Autodesk Fusion 360 part; units mm, degrees
(part 2 of 4)
  line L902 (-16.4615, 144.9808) -> (-16.4615, 149.9808)
  line L903 (-16.4615, 149.9808) -> (-20.7917, 152.4808)
  line L904 (-31.4519, 152.4808) -> (-35.782, 149.9808)
  line L905 (-35.782, 149.9808) -> (-35.782, 144.9808)
  line L906 (-35.782, 144.9808) -> (-31.4519, 142.4808)
  line L907 (-31.4519, 142.4808) -> (-27.1218, 144.9808)
  line L908 (-27.1218, 144.9808) -> (-27.1218, 149.9808)
  line L909 (-27.1218, 149.9808) -> (-31.4519, 152.4808)
  line L910 (-42.1122, 152.4808) -> (-46.4423, 149.9808)
  line L911 (-46.4423, 149.9808) -> (-46.4423, 144.9808)
  line L912 (-46.4423, 144.9808) -> (-42.1122, 142.4808)
  line L913 (-42.1122, 142.4808) -> (-37.782, 144.9808)
  line L914 (-37.782, 144.9808) -> (-37.782, 149.9808)
  line L915 (-37.782, 149.9808) -> (-42.1122, 152.4808)
  line L916 (48.5, 161.7128) -> (44.1699, 159.2128)
  line L917 (44.1699, 159.2128) -> (44.1699, 154.2128)
  line L918 (44.1699, 154.2128) -> (48.5, 151.7128)
  line L919 (48.5, 151.7128) -> (52.8301, 154.2128)
  line L920 (52.8301, 154.2128) -> (52.8301, 159.2128)
  line L921 (52.8301, 159.2128) -> (48.5, 161.7128)
  line L922 (37.8397, 161.7128) -> (33.5096, 159.2128)
  line L923 (33.5096, 159.2128) -> (33.5096, 154.2128)
  line L924 (33.5096, 154.2128) -> (37.8397, 151.7128)
  line L925 (37.8397, 151.7128) -> (42.1699, 154.2128)
  line L926 (42.1699, 154.2128) -> (42.1699, 159.2128)
  line L927 (42.1699, 159.2128) -> (37.8397, 161.7128)
  line L928 (27.1795, 161.7128) -> (22.8494, 159.2128)
  line L929 (22.8494, 159.2128) -> (22.8494, 154.2128)
  line L930 (22.8494, 154.2128) -> (27.1795, 151.7128)
  line L931 (27.1795, 151.7128) -> (31.5096, 154.2128)
  line L932 (31.5096, 154.2128) -> (31.5096, 159.2128)
  line L933 (31.5096, 159.2128) -> (27.1795, 161.7128)
  line L934 (16.5192, 161.7128) -> (12.1891, 159.2128)
  line L935 (12.1891, 159.2128) -> (12.1891, 154.2128)
  line L936 (12.1891, 154.2128) -> (16.5192, 151.7128)
  line L937 (16.5192, 151.7128) -> (20.8494, 154.2128)
  line L938 (20.8494, 154.2128) -> (20.8494, 159.2128)
  line L939 (20.8494, 159.2128) -> (16.5192, 161.7128)
  line L940 (5.859, 161.7128) -> (1.5289, 159.2128)
  line L941 (1.5289, 159.2128) -> (1.5289, 154.2128)
  line L942 (1.5289, 154.2128) -> (5.859, 151.7128)
  line L943 (5.859, 151.7128) -> (10.1891, 154.2128)
  line L944 (10.1891, 154.2128) -> (10.1891, 159.2128)
  line L945 (10.1891, 159.2128) -> (5.859, 161.7128)
  line L946 (-4.8013, 161.7128) -> (-9.1314, 159.2128)
  line L947 (-9.1314, 159.2128) -> (-9.1314, 154.2128)
  line L948 (-9.1314, 154.2128) -> (-4.8013, 151.7128)
  line L949 (-4.8013, 151.7128) -> (-0.4711, 154.2128)
  line L950 (-0.4711, 154.2128) -> (-0.4711, 159.2128)
  line L951 (-0.4711, 159.2128) -> (-4.8013, 161.7128)
  line L952 (-15.4615, 161.7128) -> (-19.7917, 159.2128)
  line L953 (-19.7917, 159.2128) -> (-19.7917, 154.2128)
  line L954 (-19.7917, 154.2128) -> (-15.4615, 151.7128)
  line L955 (-15.4615, 151.7128) -> (-11.1314, 154.2128)
  line L956 (-11.1314, 154.2128) -> (-11.1314, 159.2128)
  line L957 (-11.1314, 159.2128) -> (-15.4615, 161.7128)
  line L958 (-26.1218, 161.7128) -> (-30.4519, 159.2128)
  line L959 (-30.4519, 159.2128) -> (-30.4519, 154.2128)
  line L960 (-30.4519, 154.2128) -> (-26.1218, 151.7128)
  line L961 (-26.1218, 151.7128) -> (-21.7917, 154.2128)
  line L962 (-21.7917, 154.2128) -> (-21.7917, 159.2128)
  line L963 (-21.7917, 159.2128) -> (-26.1218, 161.7128)
  line L964 (-36.782, 161.7128) -> (-41.1122, 159.2128)
  line L965 (-41.1122, 159.2128) -> (-41.1122, 154.2128)
  line L966 (-41.1122, 154.2128) -> (-36.782, 151.7128)
  line L967 (-36.782, 151.7128) -> (-32.4519, 154.2128)
  line L968 (-32.4519, 154.2128) -> (-32.4519, 159.2128)
  line L969 (-32.4519, 159.2128) -> (-36.782, 161.7128)
  line L970 (-47.4423, 161.7128) -> (-51.7724, 159.2128)
  line L971 (-51.7724, 159.2128) -> (-51.7724, 154.2128)
  line L972 (-51.7724, 154.2128) -> (-47.4423, 151.7128)
  line L973 (-47.4423, 151.7128) -> (-43.1122, 154.2128)
  line L974 (-43.1122, 154.2128) -> (-43.1122, 159.2128)
  line L975 (-43.1122, 159.2128) -> (-47.4423, 161.7128)
  line L976 (43.1699, 170.9449) -> (38.8397, 168.4449)
  line L977 (38.8397, 168.4449) -> (38.8397, 163.4449)
  line L978 (38.8397, 163.4449) -> (43.1699, 160.9449)
  line L979 (43.1699, 160.9449) -> (47.5, 163.4449)
  line L980 (47.5, 163.4449) -> (47.5, 168.4449)
  line L981 (47.5, 168.4449) -> (43.1699, 170.9449)
  line L982 (32.5096, 170.9449) -> (28.1795, 168.4449)
  line L983 (28.1795, 168.4449) -> (28.1795, 163.4449)
  line L984 (28.1795, 163.4449) -> (32.5096, 160.9449)
  line L985 (32.5096, 160.9449) -> (36.8397, 163.4449)
  line L986 (36.8397, 163.4449) -> (36.8397, 168.4449)
  line L987 (36.8397, 168.4449) -> (32.5096, 170.9449)
  line L988 (21.8494, 170.9449) -> (17.5192, 168.4449)
  line L989 (17.5192, 168.4449) -> (17.5192, 163.4449)
  line L990 (17.5192, 163.4449) -> (21.8494, 160.9449)
  line L991 (21.8494, 160.9449) -> (26.1795, 163.4449)
  line L992 (26.1795, 163.4449) -> (26.1795, 168.4449)
  line L993 (26.1795, 168.4449) -> (21.8494, 170.9449)
  line L994 (11.1891, 170.9449) -> (6.859, 168.4449)
  line L995 (6.859, 168.4449) -> (6.859, 163.4449)
  line L996 (6.859, 163.4449) -> (11.1891, 160.9449)
  line L997 (11.1891, 160.9449) -> (15.5192, 163.4449)
  line L998 (15.5192, 163.4449) -> (15.5192, 168.4449)
  line L999 (15.5192, 168.4449) -> (11.1891, 170.9449)
  line L1000 (0.5289, 170.9449) -> (-3.8013, 168.4449)
  line L1001 (-3.8013, 168.4449) -> (-3.8013, 163.4449)
  line L1002 (-3.8013, 163.4449) -> (0.5289, 160.9449)
  line L1003 (0.5289, 160.9449) -> (4.859, 163.4449)
  line L1004 (4.859, 163.4449) -> (4.859, 168.4449)
  line L1005 (4.859, 168.4449) -> (0.5289, 170.9449)
  line L1006 (-10.1314, 170.9449) -> (-14.4615, 168.4449)
  line L1007 (-14.4615, 168.4449) -> (-14.4615, 163.4449)
  line L1008 (-14.4615, 163.4449) -> (-10.1314, 160.9449)
  line L1009 (-10.1314, 160.9449) -> (-5.8013, 163.4449)
  line L1010 (-5.8013, 163.4449) -> (-5.8013, 168.4449)
  line L1011 (-5.8013, 168.4449) -> (-10.1314, 170.9449)
  line L1012 (-20.7917, 170.9449) -> (-25.1218, 168.4449)
  line L1013 (-25.1218, 168.4449) -> (-25.1218, 163.4449)
  line L1014 (-25.1218, 163.4449) -> (-20.7917, 160.9449)
  line L1015 (-20.7917, 160.9449) -> (-16.4615, 163.4449)
  line L1016 (-16.4615, 163.4449) -> (-16.4615, 168.4449)
  line L1017 (-16.4615, 168.4449) -> (-20.7917, 170.9449)
  line L1018 (-31.4519, 170.9449) -> (-35.782, 168.4449)
  line L1019 (-35.782, 168.4449) -> (-35.782, 163.4449)
  line L1020 (-35.782, 163.4449) -> (-31.4519, 160.9449)
  line L1021 (-31.4519, 160.9449) -> (-27.1218, 163.4449)
  line L1022 (-27.1218, 163.4449) -> (-27.1218, 168.4449)
  line L1023 (-27.1218, 168.4449) -> (-31.4519, 170.9449)
  line L1024 (-42.1122, 170.9449) -> (-46.4423, 168.4449)
  line L1025 (-46.4423, 168.4449) -> (-46.4423, 163.4449)
  line L1026 (-46.4423, 163.4449) -> (-42.1122, 160.9449)
  line L1027 (-42.1122, 160.9449) -> (-37.782, 163.4449)
  line L1028 (-37.782, 163.4449) -> (-37.782, 168.4449)
  line L1029 (-37.782, 168.4449) -> (-42.1122, 170.9449)
  line L1030 (48.5, 180.1769) -> (44.1699, 177.6769)
  line L1031 (44.1699, 177.6769) -> (44.1699, 172.6769)
  line L1032 (44.1699, 172.6769) -> (48.5, 170.1769)
  line L1033 (48.5, 170.1769) -> (52.8301, 172.6769)
  line L1034 (52.8301, 172.6769) -> (52.8301, 177.6769)
  line L1035 (52.8301, 177.6769) -> (48.5, 180.1769)
  line L1036 (37.8397, 180.1769) -> (33.5096, 177.6769)
  line L1037 (33.5096, 177.6769) -> (33.5096, 172.6769)
  line L1038 (33.5096, 172.6769) -> (37.8397, 170.1769)
  line L1039 (37.8397, 170.1769) -> (42.1699, 172.6769)
  line L1040 (42.1699, 172.6769) -> (42.1699, 177.6769)
  line L1041 (42.1699, 177.6769) -> (37.8397, 180.1769)
  line L1042 (27.1795, 180.1769) -> (22.8494, 177.6769)
  line L1043 (22.8494, 177.6769) -> (22.8494, 172.6769)
  line L1044 (22.8494, 172.6769) -> (27.1795, 170.1769)
  line L1045 (27.1795, 170.1769) -> (31.5096, 172.6769)
  line L1046 (31.5096, 172.6769) -> (31.5096, 177.6769)
  line L1047 (31.5096, 177.6769) -> (27.1795, 180.1769)
  line L1048 (16.5192, 180.1769) -> (12.1891, 177.6769)
  line L1049 (12.1891, 177.6769) -> (12.1891, 172.6769)
  line L1050 (12.1891, 172.6769) -> (16.5192, 170.1769)
  line L1051 (16.5192, 170.1769) -> (20.8494, 172.6769)
  line L1052 (20.8494, 172.6769) -> (20.8494, 177.6769)
  line L1053 (20.8494, 177.6769) -> (16.5192, 180.1769)
  line L1054 (5.859, 180.1769) -> (1.5289, 177.6769)
  line L1055 (1.5289, 177.6769) -> (1.5289, 172.6769)
  line L1056 (1.5289, 172.6769) -> (5.859, 170.1769)
  line L1057 (5.859, 170.1769) -> (10.1891, 172.6769)
  line L1058 (10.1891, 172.6769) -> (10.1891, 177.6769)
  line L1059 (10.1891, 177.6769) -> (5.859, 180.1769)
  line L1060 (-4.8013, 180.1769) -> (-9.1314, 177.6769)
  line L1061 (-9.1314, 177.6769) -> (-9.1314, 172.6769)
  line L1062 (-9.1314, 172.6769) -> (-4.8013, 170.1769)
  line L1063 (-4.8013, 170.1769) -> (-0.4711, 172.6769)
  line L1064 (-0.4711, 172.6769) -> (-0.4711, 177.6769)
  line L1065 (-0.4711, 177.6769) -> (-4.8013, 180.1769)
  line L1066 (-15.4615, 180.1769) -> (-19.7917, 177.6769)
  line L1067 (-19.7917, 177.6769) -> (-19.7917, 172.6769)
  line L1068 (-19.7917, 172.6769) -> (-15.4615, 170.1769)
  line L1069 (-15.4615, 170.1769) -> (-11.1314, 172.6769)
  line L1070 (-11.1314, 172.6769) -> (-11.1314, 177.6769)
  line L1071 (-11.1314, 177.6769) -> (-15.4615, 180.1769)
  line L1072 (-26.1218, 180.1769) -> (-30.4519, 177.6769)
  line L1073 (-30.4519, 177.6769) -> (-30.4519, 172.6769)
  line L1074 (-30.4519, 172.6769) -> (-26.1218, 170.1769)
  line L1075 (-26.1218, 170.1769) -> (-21.7917, 172.6769)
  line L1076 (-21.7917, 172.6769) -> (-21.7917, 177.6769)
  line L1077 (-21.7917, 177.6769) -> (-26.1218, 180.1769)
  line L1078 (-36.782, 180.1769) -> (-41.1122, 177.6769)
  line L1079 (-41.1122, 177.6769) -> (-41.1122, 172.6769)
  line L1080 (-41.1122, 172.6769) -> (-36.782, 170.1769)
  line L1081 (-36.782, 170.1769) -> (-32.4519, 172.6769)
  line L1082 (-32.4519, 172.6769) -> (-32.4519, 177.6769)
  line L1083 (-32.4519, 177.6769) -> (-36.782, 180.1769)
  line L1084 (-47.4423, 180.1769) -> (-51.7724, 177.6769)
  line L1085 (-51.7724, 177.6769) -> (-51.7724, 172.6769)
  line L1086 (-51.7724, 172.6769) -> (-47.4423, 170.1769)
  line L1087 (-47.4423, 170.1769) -> (-43.1122, 172.6769)
  line L1088 (-43.1122, 172.6769) -> (-43.1122, 177.6769)
  line L1089 (-43.1122, 177.6769) -> (-47.4423, 180.1769)
  line L1090 (43.1699, 189.409) -> (38.8397, 186.909)
  line L1091 (38.8397, 186.909) -> (38.8397, 181.909)
  line L1092 (38.8397, 181.909) -> (43.1699, 179.409)
  line L1093 (43.1699, 179.409) -> (47.5, 181.909)
  line L1094 (47.5, 181.909) -> (47.5, 186.909)
  line L1095 (47.5, 186.909) -> (43.1699, 189.409)
  line L1096 (32.5096, 189.409) -> (28.1795, 186.909)
  line L1097 (28.1795, 186.909) -> (28.1795, 181.909)
  line L1098 (28.1795, 181.909) -> (32.5096, 179.409)
  line L1099 (32.5096, 179.409) -> (36.8397, 181.909)
  line L1100 (36.8397, 181.909) -> (36.8397, 186.909)
  line L1101 (36.8397, 186.909) -> (32.5096, 189.409)
  line L1102 (21.8494, 189.409) -> (17.5192, 186.909)
  line L1103 (17.5192, 186.909) -> (17.5192, 181.909)
  line L1104 (17.5192, 181.909) -> (21.8494, 179.409)
  line L1105 (21.8494, 179.409) -> (26.1795, 181.909)
  line L1106 (26.1795, 181.909) -> (26.1795, 186.909)
  line L1107 (26.1795, 186.909) -> (21.8494, 189.409)
  line L1108 (11.1891, 189.409) -> (6.859, 186.909)
  line L1109 (6.859, 186.909) -> (6.859, 181.909)
  line L1110 (6.859, 181.909) -> (11.1891, 179.409)
  line L1111 (11.1891, 179.409) -> (15.5192, 181.909)
  line L1112 (15.5192, 181.909) -> (15.5192, 186.909)
  line L1113 (15.5192, 186.909) -> (11.1891, 189.409)
  line L1114 (0.5289, 189.409) -> (-3.8013, 186.909)
  line L1115 (-3.8013, 186.909) -> (-3.8013, 181.909)
  line L1116 (-3.8013, 181.909) -> (0.5289, 179.409)
  line L1117 (0.5289, 179.409) -> (4.859, 181.909)
  line L1118 (4.859, 181.909) -> (4.859, 186.909)
  line L1119 (4.859, 186.909) -> (0.5289, 189.409)
  line L1120 (-10.1314, 189.409) -> (-14.4615, 186.909)
  line L1121 (-14.4615, 186.909) -> (-14.4615, 181.909)
  line L1122 (-14.4615, 181.909) -> (-10.1314, 179.409)
  line L1123 (-10.1314, 179.409) -> (-5.8013, 181.909)
  line L1124 (-5.8013, 181.909) -> (-5.8013, 186.909)
  line L1125 (-5.8013, 186.909) -> (-10.1314, 189.409)
  line L1126 (-20.7917, 189.409) -> (-25.1218, 186.909)
  line L1127 (-25.1218, 186.909) -> (-25.1218, 181.909)
  line L1128 (-25.1218, 181.909) -> (-20.7917, 179.409)
  line L1129 (-20.7917, 179.409) -> (-16.4615, 181.909)
  line L1130 (-16.4615, 181.909) -> (-16.4615, 186.909)
  line L1131 (-16.4615, 186.909) -> (-20.7917, 189.409)
  line L1132 (-31.4519, 189.409) -> (-35.782, 186.909)
  line L1133 (-35.782, 186.909) -> (-35.782, 181.909)
  line L1134 (-35.782, 181.909) -> (-31.4519, 179.409)
  line L1135 (-31.4519, 179.409) -> (-27.1218, 181.909)
  line L1136 (-27.1218, 181.909) -> (-27.1218, 186.909)
  line L1137 (-27.1218, 186.909) -> (-31.4519, 189.409)
  line L1138 (-42.1122, 189.409) -> (-46.4423, 186.909)
  line L1139 (-46.4423, 186.909) -> (-46.4423, 181.909)
  line L1140 (-46.4423, 181.909) -> (-42.1122, 179.409)
  line L1141 (-42.1122, 179.409) -> (-37.782, 181.909)
  line L1142 (-37.782, 181.909) -> (-37.782, 186.909)
  line L1143 (-37.782, 186.909) -> (-42.1122, 189.409)
  line L1144 (48.5, 198.641) -> (44.1699, 196.141)
  line L1145 (44.1699, 196.141) -> (44.1699, 191.141)
  line L1146 (44.1699, 191.141) -> (48.5, 188.641)
  line L1147 (48.5, 188.641) -> (52.8301, 191.141)
  line L1148 (52.8301, 191.141) -> (52.8301, 196.141)
  line L1149 (52.8301, 196.141) -> (48.5, 198.641)
  line L1150 (37.8397, 198.641) -> (33.5096, 196.141)
  line L1151 (33.5096, 196.141) -> (33.5096, 191.141)
  line L1152 (33.5096, 191.141) -> (37.8397, 188.641)
  line L1153 (37.8397, 188.641) -> (42.1699, 191.141)
  line L1154 (42.1699, 191.141) -> (42.1699, 196.141)
  line L1155 (42.1699, 196.141) -> (37.8397, 198.641)
  line L1156 (27.1795, 198.641) -> (22.8494, 196.141)
  line L1157 (22.8494, 196.141) -> (22.8494, 191.141)
  line L1158 (22.8494, 191.141) -> (27.1795, 188.641)
  line L1159 (27.1795, 188.641) -> (31.5096, 191.141)
  line L1160 (31.5096, 191.141) -> (31.5096, 196.141)
  line L1161 (31.5096, 196.141) -> (27.1795, 198.641)
  line L1162 (16.5192, 198.641) -> (12.1891, 196.141)
  line L1163 (12.1891, 196.141) -> (12.1891, 191.141)
  line L1164 (12.1891, 191.141) -> (16.5192, 188.641)
  line L1165 (16.5192, 188.641) -> (20.8494, 191.141)
  line L1166 (20.8494, 191.141) -> (20.8494, 196.141)
  line L1167 (20.8494, 196.141) -> (16.5192, 198.641)
  line L1168 (5.859, 198.641) -> (1.5289, 196.141)
  line L1169 (1.5289, 196.141) -> (1.5289, 191.141)
  line L1170 (1.5289, 191.141) -> (5.859, 188.641)
  line L1171 (5.859, 188.641) -> (10.1891, 191.141)
  line L1172 (10.1891, 191.141) -> (10.1891, 196.141)
  line L1173 (10.1891, 196.141) -> (5.859, 198.641)
  line L1174 (-4.8013, 198.641) -> (-9.1314, 196.141)
  line L1175 (-9.1314, 196.141) -> (-9.1314, 191.141)
  line L1176 (-9.1314, 191.141) -> (-4.8013, 188.641)
  line L1177 (-4.8013, 188.641) -> (-0.4711, 191.141)
  line L1178 (-0.4711, 191.141) -> (-0.4711, 196.141)
  line L1179 (-0.4711, 196.141) -> (-4.8013, 198.641)
  line L1180 (-15.4615, 198.641) -> (-19.7917, 196.141)
  line L1181 (-19.7917, 196.141) -> (-19.7917, 191.141)
  line L1182 (-19.7917, 191.141) -> (-15.4615, 188.641)
  line L1183 (-15.4615, 188.641) -> (-11.1314, 191.141)
  line L1184 (-11.1314, 191.141) -> (-11.1314, 196.141)
  line L1185 (-11.1314, 196.141) -> (-15.4615, 198.641)
  line L1186 (-26.1218, 198.641) -> (-30.4519, 196.141)
  line L1187 (-30.4519, 196.141) -> (-30.4519, 191.141)
  line L1188 (-30.4519, 191.141) -> (-26.1218, 188.641)
  line L1189 (-26.1218, 188.641) -> (-21.7917, 191.141)
  line L1190 (-21.7917, 191.141) -> (-21.7917, 196.141)
  line L1191 (-21.7917, 196.141) -> (-26.1218, 198.641)
  line L1192 (-36.782, 198.641) -> (-41.1122, 196.141)
  line L1193 (-41.1122, 196.141) -> (-41.1122, 191.141)
  line L1194 (-41.1122, 191.141) -> (-36.782, 188.641)
  line L1195 (-36.782, 188.641) -> (-32.4519, 191.141)
  line L1196 (-32.4519, 191.141) -> (-32.4519, 196.141)
  line L1197 (-32.4519, 196.141) -> (-36.782, 198.641)
  line L1198 (-47.4423, 198.641) -> (-51.7724, 196.141)
  line L1199 (-51.7724, 196.141) -> (-51.7724, 191.141)
  line L1200 (-51.7724, 191.141) -> (-47.4423, 188.641)
  line L1201 (-47.4423, 188.641) -> (-43.1122, 191.141)
  line L1202 (-43.1122, 191.141) -> (-43.1122, 196.141)
  line L1203 (-43.1122, 196.141) -> (-47.4423, 198.641)
  line L1204 (43.1699, 207.8731) -> (38.8397, 205.3731)
  line L1205 (38.8397, 205.3731) -> (38.8397, 200.3731)
  line L1206 (38.8397, 200.3731) -> (43.1699, 197.8731)
  line L1207 (43.1699, 197.8731) -> (47.5, 200.3731)
  line L1208 (47.5, 200.3731) -> (47.5, 205.3731)
  line L1209 (47.5, 205.3731) -> (43.1699, 207.8731)
  line L1210 (32.5096, 207.8731) -> (28.1795, 205.3731)
  line L1211 (28.1795, 205.3731) -> (28.1795, 200.3731)
  line L1212 (28.1795, 200.3731) -> (32.5096, 197.8731)
  line L1213 (32.5096, 197.8731) -> (36.8397, 200.3731)
  line L1214 (36.8397, 200.3731) -> (36.8397, 205.3731)
  line L1215 (36.8397, 205.3731) -> (32.5096, 207.8731)
  line L1216 (21.8494, 207.8731) -> (17.5192, 205.3731)
  line L1217 (17.5192, 205.3731) -> (17.5192, 200.3731)
  line L1218 (17.5192, 200.3731) -> (21.8494, 197.8731)
  line L1219 (21.8494, 197.8731) -> (26.1795, 200.3731)
  line L1220 (26.1795, 200.3731) -> (26.1795, 205.3731)
  line L1221 (26.1795, 205.3731) -> (21.8494, 207.8731)
  line L1222 (11.1891, 207.8731) -> (6.859, 205.3731)
  line L1223 (6.859, 205.3731) -> (6.859, 200.3731)
  line L1224 (6.859, 200.3731) -> (11.1891, 197.8731)
  line L1225 (11.1891, 197.8731) -> (15.5192, 200.3731)
  line L1226 (15.5192, 200.3731) -> (15.5192, 205.3731)
  line L1227 (15.5192, 205.3731) -> (11.1891, 207.8731)
  line L1228 (0.5289, 207.8731) -> (-3.8013, 205.3731)
  line L1229 (-3.8013, 205.3731) -> (-3.8013, 200.3731)
  line L1230 (-3.8013, 200.3731) -> (0.5289, 197.8731)
  line L1231 (0.5289, 197.8731) -> (4.859, 200.3731)
  line L1232 (4.859, 200.3731) -> (4.859, 205.3731)
  line L1233 (4.859, 205.3731) -> (0.5289, 207.8731)
  line L1234 (-10.1314, 207.8731) -> (-14.4615, 205.3731)
  line L1235 (-14.4615, 205.3731) -> (-14.4615, 200.3731)
  line L1236 (-14.4615, 200.3731) -> (-10.1314, 197.8731)
  line L1237 (-10.1314, 197.8731) -> (-5.8013, 200.3731)
  line L1238 (-5.8013, 200.3731) -> (-5.8013, 205.3731)
  line L1239 (-5.8013, 205.3731) -> (-10.1314, 207.8731)
  line L1240 (-20.7917, 207.8731) -> (-25.1218, 205.3731)
  line L1241 (-25.1218, 205.3731) -> (-25.1218, 200.3731)
  line L1242 (-25.1218, 200.3731) -> (-20.7917, 197.8731)
  line L1243 (-20.7917, 197.8731) -> (-16.4615, 200.3731)
  line L1244 (-16.4615, 200.3731) -> (-16.4615, 205.3731)
  line L1245 (-16.4615, 205.3731) -> (-20.7917, 207.8731)
  line L1246 (-31.4519, 207.8731) -> (-35.782, 205.3731)
  line L1247 (-35.782, 205.3731) -> (-35.782, 200.3731)
  line L1248 (-35.782, 200.3731) -> (-31.4519, 197.8731)
  line L1249 (-31.4519, 197.8731) -> (-27.1218, 200.3731)
  line L1250 (-27.1218, 200.3731) -> (-27.1218, 205.3731)
  line L1251 (-27.1218, 205.3731) -> (-31.4519, 207.8731)
  line L1252 (-42.1122, 207.8731) -> (-46.4423, 205.3731)
  line L1253 (-46.4423, 205.3731) -> (-46.4423, 200.3731)
  line L1254 (-46.4423, 200.3731) -> (-42.1122, 197.8731)
  line L1255 (-42.1122, 197.8731) -> (-37.782, 200.3731)
  line L1256 (-37.782, 200.3731) -> (-37.782, 205.3731)
  line L1257 (-37.782, 205.3731) -> (-42.1122, 207.8731)
  line L1258 (48.5, 217.1051) -> (44.1699, 214.6051)
  line L1259 (44.1699, 214.6051) -> (44.1699, 209.6051)
  line L1260 (44.1699, 209.6051) -> (48.5, 207.1051)
  line L1261 (48.5, 207.1051) -> (52.8301, 209.6051)
  line L1262 (52.8301, 209.6051) -> (52.8301, 214.6051)
  line L1263 (52.8301, 214.6051) -> (48.5, 217.1051)
  line L1264 (37.8397, 217.1051) -> (33.5096, 214.6051)
  line L1265 (33.5096, 214.6051) -> (33.5096, 209.6051)
  line L1266 (33.5096, 209.6051) -> (37.8397, 207.1051)
  line L1267 (37.8397, 207.1051) -> (42.1699, 209.6051)
  line L1268 (42.1699, 209.6051) -> (42.1699, 214.6051)
  line L1269 (42.1699, 214.6051) -> (37.8397, 217.1051)
  line L1270 (27.1795, 217.1051) -> (22.8494, 214.6051)
  line L1271 (22.8494, 214.6051) -> (22.8494, 209.6051)
  line L1272 (22.8494, 209.6051) -> (27.1795, 207.1051)
  line L1273 (27.1795, 207.1051) -> (31.5096, 209.6051)
  line L1274 (31.5096, 209.6051) -> (31.5096, 214.6051)
  line L1275 (31.5096, 214.6051) -> (27.1795, 217.1051)
  line L1276 (16.5192, 217.1051) -> (12.1891, 214.6051)
  line L1277 (12.1891, 214.6051) -> (12.1891, 209.6051)
  line L1278 (12.1891, 209.6051) -> (16.5192, 207.1051)
  line L1279 (16.5192, 207.1051) -> (20.8494, 209.6051)
  line L1280 (20.8494, 209.6051) -> (20.8494, 214.6051)
  line L1281 (20.8494, 214.6051) -> (16.5192, 217.1051)
  line L1282 (5.859, 217.1051) -> (1.5289, 214.6051)
  line L1283 (1.5289, 214.6051) -> (1.5289, 209.6051)
  line L1284 (1.5289, 209.6051) -> (5.859, 207.1051)
  line L1285 (5.859, 207.1051) -> (10.1891, 209.6051)
  line L1286 (10.1891, 209.6051) -> (10.1891, 214.6051)
  line L1287 (10.1891, 214.6051) -> (5.859, 217.1051)
  line L1288 (-4.8013, 217.1051) -> (-9.1314, 214.6051)
  line L1289 (-9.1314, 214.6051) -> (-9.1314, 209.6051)
  line L1290 (-9.1314, 209.6051) -> (-4.8013, 207.1051)
  line L1291 (-4.8013, 207.1051) -> (-0.4711, 209.6051)
  line L1292 (-0.4711, 209.6051) -> (-0.4711, 214.6051)
  line L1293 (-0.4711, 214.6051) -> (-4.8013, 217.1051)
  line L1294 (-15.4615, 217.1051) -> (-19.7917, 214.6051)
  line L1295 (-19.7917, 214.6051) -> (-19.7917, 209.6051)
  line L1296 (-19.7917, 209.6051) -> (-15.4615, 207.1051)
  line L1297 (-15.4615, 207.1051) -> (-11.1314, 209.6051)
  line L1298 (-11.1314, 209.6051) -> (-11.1314, 214.6051)
  line L1299 (-11.1314, 214.6051) -> (-15.4615, 217.1051)
  line L1300 (-26.1218, 217.1051) -> (-30.4519, 214.6051)
  line L1301 (-30.4519, 214.6051) -> (-30.4519, 209.6051)
  line L1302 (-30.4519, 209.6051) -> (-26.1218, 207.1051)
  line L1303 (-26.1218, 207.1051) -> (-21.7917, 209.6051)
  line L1304 (-21.7917, 209.6051) -> (-21.7917, 214.6051)
  line L1305 (-21.7917, 214.6051) -> (-26.1218, 217.1051)
  line L1306 (-36.782, 217.1051) -> (-41.1122, 214.6051)
  line L1307 (-41.1122, 214.6051) -> (-41.1122, 209.6051)
  line L1308 (-41.1122, 209.6051) -> (-36.782, 207.1051)
  line L1309 (-36.782, 207.1051) -> (-32.4519, 209.6051)
  line L1310 (-32.4519, 209.6051) -> (-32.4519, 214.6051)
  line L1311 (-32.4519, 214.6051) -> (-36.782, 217.1051)
  line L1312 (-47.4423, 217.1051) -> (-51.7724, 214.6051)
  line L1313 (-51.7724, 214.6051) -> (-51.7724, 209.6051)
  line L1314 (-51.7724, 209.6051) -> (-47.4423, 207.1051)
  line L1315 (-47.4423, 207.1051) -> (-43.1122, 209.6051)
  line L1316 (-43.1122, 209.6051) -> (-43.1122, 214.6051)
  line L1317 (-43.1122, 214.6051) -> (-47.4423, 217.1051)
  line L1318 (43.1699, 226.3372) -> (38.8397, 223.8372)
  line L1319 (38.8397, 223.8372) -> (38.8397, 218.8372)
  line L1320 (38.8397, 218.8372) -> (43.1699, 216.3372)
  line L1321 (43.1699, 216.3372) -> (47.5, 218.8372)
  line L1322 (47.5, 218.8372) -> (47.5, 223.8372)
  line L1323 (47.5, 223.8372) -> (43.1699, 226.3372)
  line L1324 (32.5096, 226.3372) -> (28.1795, 223.8372)
  line L1325 (28.1795, 223.8372) -> (28.1795, 218.8372)
  line L1326 (28.1795, 218.8372) -> (32.5096, 216.3372)
  line L1327 (32.5096, 216.3372) -> (36.8397, 218.8372)
  line L1328 (36.8397, 218.8372) -> (36.8397, 223.8372)
  line L1329 (36.8397, 223.8372) -> (32.5096, 226.3372)
  line L1330 (21.8494, 226.3372) -> (17.5192, 223.8372)
  line L1331 (17.5192, 223.8372) -> (17.5192, 218.8372)
  line L1332 (17.5192, 218.8372) -> (21.8494, 216.3372)
  line L1333 (21.8494, 216.3372) -> (26.1795, 218.8372)
  line L1334 (26.1795, 218.8372) -> (26.1795, 223.8372)
  line L1335 (26.1795, 223.8372) -> (21.8494, 226.3372)
  line L1336 (11.1891, 226.3372) -> (6.859, 223.8372)
  line L1337 (6.859, 223.8372) -> (6.859, 218.8372)
  line L1338 (6.859, 218.8372) -> (11.1891, 216.3372)
  line L1339 (11.1891, 216.3372) -> (15.5192, 218.8372)
  line L1340 (15.5192, 218.8372) -> (15.5192, 223.8372)
  line L1341 (15.5192, 223.8372) -> (11.1891, 226.3372)
  line L1342 (0.5289, 226.3372) -> (-3.8013, 223.8372)
  line L1343 (-3.8013, 223.8372) -> (-3.8013, 218.8372)
  line L1344 (-3.8013, 218.8372) -> (0.5289, 216.3372)
  line L1345 (0.5289, 216.3372) -> (4.859, 218.8372)
  line L1346 (4.859, 218.8372) -> (4.859, 223.8372)
  line L1347 (4.859, 223.8372) -> (0.5289, 226.3372)
  line L1348 (-10.1314, 226.3372) -> (-14.4615, 223.8372)
  line L1349 (-14.4615, 223.8372) -> (-14.4615, 218.8372)
  line L1350 (-14.4615, 218.8372) -> (-10.1314, 216.3372)
  line L1351 (-10.1314, 216.3372) -> (-5.8013, 218.8372)
  line L1352 (-5.8013, 218.8372) -> (-5.8013, 223.8372)
  line L1353 (-5.8013, 223.8372) -> (-10.1314, 226.3372)
  line L1354 (-20.7917, 226.3372) -> (-25.1218, 223.8372)
  line L1355 (-25.1218, 223.8372) -> (-25.1218, 218.8372)
  line L1356 (-25.1218, 218.8372) -> (-20.7917, 216.3372)
  line L1357 (-20.7917, 216.3372) -> (-16.4615, 218.8372)
  line L1358 (-16.4615, 218.8372) -> (-16.4615, 223.8372)
  line L1359 (-16.4615, 223.8372) -> (-20.7917, 226.3372)
  line L1360 (-31.4519, 226.3372) -> (-35.782, 223.8372)
  line L1361 (-35.782, 223.8372) -> (-35.782, 218.8372)
  line L1362 (-35.782, 218.8372) -> (-31.4519, 216.3372)
  line L1363 (-31.4519, 216.3372) -> (-27.1218, 218.8372)
  line L1364 (-27.1218, 218.8372) -> (-27.1218, 223.8372)
  line L1365 (-27.1218, 223.8372) -> (-31.4519, 226.3372)
  line L1366 (-42.1122, 226.3372) -> (-46.4423, 223.8372)
  line L1367 (-46.4423, 223.8372) -> (-46.4423, 218.8372)
  line L1368 (-46.4423, 218.8372) -> (-42.1122, 216.3372)
  line L1369 (-42.1122, 216.3372) -> (-37.782, 218.8372)
  line L1370 (-37.782, 218.8372) -> (-37.782, 223.8372)
  line L1371 (-37.782, 223.8372) -> (-42.1122, 226.3372)
  line L1372 (48.5, 235.5692) -> (44.1699, 233.0692)
  line L1373 (44.1699, 233.0692) -> (44.1699, 228.0692)
  line L1374 (44.1699, 228.0692) -> (48.5, 225.5692)
  line L1375 (48.5, 225.5692) -> (52.8301, 228.0692)
  line L1376 (52.8301, 228.0692) -> (52.8301, 233.0692)
  line L1377 (52.8301, 233.0692) -> (48.5, 235.5692)
  line L1378 (37.8397, 235.5692) -> (33.5096, 233.0692)
  line L1379 (33.5096, 233.0692) -> (33.5096, 228.0692)
  line L1380 (33.5096, 228.0692) -> (37.8397, 225.5692)
  line L1381 (37.8397, 225.5692) -> (42.1699, 228.0692)
  line L1382 (42.1699, 228.0692) -> (42.1699, 233.0692)
  line L1383 (42.1699, 233.0692) -> (37.8397, 235.5692)
  line L1384 (27.1795, 235.5692) -> (22.8494, 233.0692)
  line L1385 (22.8494, 233.0692) -> (22.8494, 228.0692)
  line L1386 (22.8494, 228.0692) -> (27.1795, 225.5692)
  line L1387 (27.1795, 225.5692) -> (31.5096, 228.0692)
  line L1388 (31.5096, 228.0692) -> (31.5096, 233.0692)
  line L1389 (31.5096, 233.0692) -> (27.1795, 235.5692)
  line L1390 (16.5192, 235.5692) -> (12.1891, 233.0692)
  line L1391 (12.1891, 233.0692) -> (12.1891, 228.0692)
  line L1392 (12.1891, 228.0692) -> (16.5192, 225.5692)
  line L1393 (16.5192, 225.5692) -> (20.8494, 228.0692)
  line L1394 (20.8494, 228.0692) -> (20.8494, 233.0692)
  line L1395 (20.8494, 233.0692) -> (16.5192, 235.5692)
  line L1396 (5.859, 235.5692) -> (1.5289, 233.0692)
  line L1397 (1.5289, 233.0692) -> (1.5289, 228.0692)
  line L1398 (1.5289, 228.0692) -> (5.859, 225.5692)
  line L1399 (5.859, 225.5692) -> (10.1891, 228.0692)
  line L1400 (10.1891, 228.0692) -> (10.1891, 233.0692)
  line L1401 (10.1891, 233.0692) -> (5.859, 235.5692)
  line L1402 (-4.8013, 235.5692) -> (-9.1314, 233.0692)
  line L1403 (-9.1314, 233.0692) -> (-9.1314, 228.0692)
  line L1404 (-9.1314, 228.0692) -> (-4.8013, 225.5692)
  line L1405 (-4.8013, 225.5692) -> (-0.4711, 228.0692)
  line L1406 (-0.4711, 228.0692) -> (-0.4711, 233.0692)
  line L1407 (-0.4711, 233.0692) -> (-4.8013, 235.5692)
  line L1408 (-15.4615, 235.5692) -> (-19.7917, 233.0692)
  line L1409 (-19.7917, 233.0692) -> (-19.7917, 228.0692)
  line L1410 (-19.7917, 228.0692) -> (-15.4615, 225.5692)
  line L1411 (-15.4615, 225.5692) -> (-11.1314, 228.0692)
  line L1412 (-11.1314, 228.0692) -> (-11.1314, 233.0692)
  line L1413 (-11.1314, 233.0692) -> (-15.4615, 235.5692)
  line L1414 (-26.1218, 235.5692) -> (-30.4519, 233.0692)
  line L1415 (-30.4519, 233.0692) -> (-30.4519, 228.0692)
  line L1416 (-30.4519, 228.0692) -> (-26.1218, 225.5692)
  line L1417 (-26.1218, 225.5692) -> (-21.7917, 228.0692)
  line L1418 (-21.7917, 228.0692) -> (-21.7917, 233.0692)
  line L1419 (-21.7917, 233.0692) -> (-26.1218, 235.5692)
  line L1420 (-36.782, 235.5692) -> (-41.1122, 233.0692)
  line L1421 (-41.1122, 233.0692) -> (-41.1122, 228.0692)
  line L1422 (-41.1122, 228.0692) -> (-36.782, 225.5692)
  line L1423 (-36.782, 225.5692) -> (-32.4519, 228.0692)
  line L1424 (-32.4519, 228.0692) -> (-32.4519, 233.0692)
  line L1425 (-32.4519, 233.0692) -> (-36.782, 235.5692)
  line L1426 (-47.4423, 235.5692) -> (-51.7724, 233.0692)
  line L1427 (-51.7724, 233.0692) -> (-51.7724, 228.0692)
  line L1428 (-51.7724, 228.0692) -> (-47.4423, 225.5692)
  line L1429 (-47.4423, 225.5692) -> (-43.1122, 228.0692)
  line L1430 (-43.1122, 228.0692) -> (-43.1122, 233.0692)
  line L1431 (-43.1122, 233.0692) -> (-47.4423, 235.5692)
  line L1432 (43.1699, 244.8013) -> (38.8397, 242.3013)
  line L1433 (38.8397, 242.3013) -> (38.8397, 237.3013)
  line L1434 (38.8397, 237.3013) -> (43.1699, 234.8013)
  line L1435 (43.1699, 234.8013) -> (47.5, 237.3013)
  line L1436 (47.5, 237.3013) -> (47.5, 242.3013)
  line L1437 (47.5, 242.3013) -> (43.1699, 244.8013)
  line L1438 (32.5096, 244.8013) -> (28.1795, 242.3013)
  line L1439 (28.1795, 242.3013) -> (28.1795, 237.3013)
  line L1440 (28.1795, 237.3013) -> (32.5096, 234.8013)
  line L1441 (32.5096, 234.8013) -> (36.8397, 237.3013)
  line L1442 (36.8397, 237.3013) -> (36.8397, 242.3013)
  line L1443 (36.8397, 242.3013) -> (32.5096, 244.8013)
  line L1444 (21.8494, 244.8013) -> (17.5192, 242.3013)
  line L1445 (17.5192, 242.3013) -> (17.5192, 237.3013)
  line L1446 (17.5192, 237.3013) -> (21.8494, 234.8013)
  line L1447 (21.8494, 234.8013) -> (26.1795, 237.3013)
  line L1448 (26.1795, 237.3013) -> (26.1795, 242.3013)
  line L1449 (26.1795, 242.3013) -> (21.8494, 244.8013)
  line L1450 (11.1891, 244.8013) -> (6.859, 242.3013)
  line L1451 (6.859, 242.3013) -> (6.859, 237.3013)
  line L1452 (6.859, 237.3013) -> (11.1891, 234.8013)
  line L1453 (11.1891, 234.8013) -> (15.5192, 237.3013)
  line L1454 (15.5192, 237.3013) -> (15.5192, 242.3013)
  line L1455 (15.5192, 242.3013) -> (11.1891, 244.8013)
  line L1456 (0.5289, 244.8013) -> (-3.8013, 242.3013)
  line L1457 (-3.8013, 242.3013) -> (-3.8013, 237.3013)
  line L1458 (-3.8013, 237.3013) -> (0.5289, 234.8013)
  line L1459 (0.5289, 234.8013) -> (4.859, 237.3013)
  line L1460 (4.859, 237.3013) -> (4.859, 242.3013)
  line L1461 (4.859, 242.3013) -> (0.5289, 244.8013)
  line L1462 (-10.1314, 244.8013) -> (-14.4615, 242.3013)
  line L1463 (-14.4615, 242.3013) -> (-14.4615, 237.3013)
  line L1464 (-14.4615, 237.3013) -> (-10.1314, 234.8013)
  line L1465 (-10.1314, 234.8013) -> (-5.8013, 237.3013)
  line L1466 (-5.8013, 237.3013) -> (-5.8013, 242.3013)
  line L1467 (-5.8013, 242.3013) -> (-10.1314, 244.8013)
  line L1468 (-20.7917, 244.8013) -> (-25.1218, 242.3013)
  line L1469 (-25.1218, 242.3013) -> (-25.1218, 237.3013)
  line L1470 (-25.1218, 237.3013) -> (-20.7917, 234.8013)
  line L1471 (-20.7917, 234.8013) -> (-16.4615, 237.3013)
  line L1472 (-16.4615, 237.3013) -> (-16.4615, 242.3013)
  line L1473 (-16.4615, 242.3013) -> (-20.7917, 244.8013)
  line L1474 (-31.4519, 244.8013) -> (-35.782, 242.3013)
  line L1475 (-35.782, 242.3013) -> (-35.782, 237.3013)
  line L1476 (-35.782, 237.3013) -> (-31.4519, 234.8013)
  line L1477 (-31.4519, 234.8013) -> (-27.1218, 237.3013)
  line L1478 (-27.1218, 237.3013) -> (-27.1218, 242.3013)
  line L1479 (-27.1218, 242.3013) -> (-31.4519, 244.8013)
  line L1480 (-42.1122, 244.8013) -> (-46.4423, 242.3013)
  line L1481 (-46.4423, 242.3013) -> (-46.4423, 237.3013)
  line L1482 (-46.4423, 237.3013) -> (-42.1122, 234.8013)
  line L1483 (-42.1122, 234.8013) -> (-37.782, 237.3013)
  line L1484 (-37.782, 237.3013) -> (-37.782, 242.3013)
  line L1485 (-37.782, 242.3013) -> (-42.1122, 244.8013)
extrude "拉伸4" cut sketch "草图4" against normal blind 4 contours L4 L5 L6 L7 L8 L9 | L10 L11 L12 L13 L14 L15 | L16 L17 L18 L19 L20 L21 | L22 L23 L24 L25 L26 L27 | L28 L29 L30 L31 L32 L33 | L34 L35 L36 L37 L38 L39 | L40 L41 L42 L43 L44 L45 | L46 L47 L48 L49 L50 L51 | L52 L53 L54 L55 L56 L57 | L58 L59 L60 L61 L62 L63 | L64 L65 L66 L67 L68 L69 | L70 L71 L72 L73 L74 L75 | L76 L77 L78 L79 L80 L81 | L82 L83 L84 L85 L86 L87 | L88 L89 L90 L91 L92 L93 | L94 L95 L96 L97 L98 L99 | L100 L101 L102 L103 L104 L105 | L106 L107 L108 L109 L110 L111 | L112 L113 L114 L115 L116 L117 | L118 L119 L120 L121 L122 L123 | L124 L125 L126 L127 L128 L129 | L130 L131 L132 L133 L134 L135 | L136 L137 L138 L139 L140 L141 | L142 L143 L144 L145 L146 L147 | L148 L149 L150 L151 L152 L153 | L154 L155 L156 L157 L158 L159 | L160 L161 L162 L163 L164 L165 | L166 L167 L168 L169 L170 L171 | L172 L173 L174 L175 L176 L177 | L178 L179 L180 L181 L182 L183 | L184 L185 L186 L187 L188 L189 | L190 L191 L192 L193 L194 L195 | L196 L197 L198 L199 L200 L201 | L202 L203 L204 L205 L206 L207 | L208 L209 L210 L211 L212 L213 | L214 L215 L216 L217 L218 L219 | L220 L221 L222 L223 L224 L225 | L226 L227 L228 L229 L230 L231 | L232 L233 L234 L235 L236 L237 | L238 L239 L240 L241 L242 L243 | L244 L245 L246 L247 L248 L249 | L250 L251 L252 L253 L254 L255 | L256 L257 L258 L259 L260 L261 | L262 L263 L264 L265 L266 L267 | L268 L269 L270 L271 L272 L273 | L274 L275 L276 L277 L278 L279 | L280 L281 L282 L283 L284 L285 | L286 L287 L288 L289 L290 L291 | L292 L293 L294 L295 L296 L297 | L298 L299 L300 L301 L302 L303 | L304 L305 L306 L307 L308 L309 | L310 L311 L312 L313 L314 L315 | L316 L317 L318 L319 L320 L321 | L322 L323 L324 L325 L326 L327 | L328 L329 L330 L331 L332 L333 | L334 L335 L336 L337 L338 L339 | L340 L341 L342 L343 L344 L345 | L346 L347 L348 L349 L350 L351 | L352 L353 L354 L355 L356 L357 | L358 L359 L360 L361 L362 L363 | L364 L365 L366 L367 L368 L369 | L370 L371 L372 L373 L374 L375 | L376 L377 L378 L379 L380 L381 | L382 L383 L384 L385 L386 L387 | L388 L389 L390 L391 L392 L393 | L394 L395 L396 L397 L398 L399 | L400 L401 L402 L403 L404 L405 | L406 L407 L408 L409 L410 L411 | L412 L413 L414 L415 L416 L417 | L418 L419 L420 L421 L422 L423 | L424 L425 L426 L427 L428 L429 | L430 L431 L432 L433 L434 L435 | L436 L437 L438 L439 L440 L441 | L442 L443 L444 L445 L446 L447 | L448 L449 L450 L451 L452 L453 | L454 L455 L456 L457 L458 L459 | L460 L461 L462 L463 L464 L465 | L466 L467 L468 L469 L470 L471 | L472 L473 L474 L475 L476 L477 | L478 L479 L480 L481 L482 L483 | L484 L485 L486 L487 L488 L489 | L490 L491 L492 L493 L494 L495 | L496 L497 L498 L499 L500 L501 | L502 L503 L504 L505 L506 L507 | L508 L509 L510 L511 L512 L513 | L514 L515 L516 L517 L518 L519 | L520 L521 L522 L523 L524 L525 | L526 L527 L528 L529 L530 L531 | L532 L533 L534 L535 L536 L537 | L538 L539 L540 L541 L542 L543 | L544 L545 L546 L547 L548 L549 | L550 L551 L552 L553 L554 L555 | L556 L557 L558 L559 L560 L561 | L562 L563 L564 L565 L566 L567 | L568 L569 L570 L571 L572 L573 | L574 L575 L576 L577 L578 L579 | L580 L581 L582 L583 L584 L585 | L586 L587 L588 L589 L590 L591 | L592 L593 L594 L595 L596 L597 | L598 L599 L600 L601 L602 L603 | L604 L605 L606 L607 L608 L609 | L610 L611 L612 L613 L614 L615 | L616 L617 L618 L619 L620 L621 | L622 L623 L624 L625 L626 L627 | L628 L629 L630 L631 L632 L633 | L634 L635 L636 L637 L638 L639 | L640 L641 L642 L643 L644 L645 | L646 L647 L648 L649 L650 L651 | L652 L653 L654 L655 L656 L657 | L658 L659 L660 L661 L662 L663 | L664 L665 L666 L667 L668 L669 | L670 L671 L672 L673 L674 L675 | L676 L677 L678 L679 L680 L681 | L682 L683 L684 L685 L686 L687 | L688 L689 L690 L691 L692 L693 | L694 L695 L696 L697 L698 L699 | L700 L701 L702 L703 L704 L705 | L706 L707 L708 L709 L710 L711 | L712 L713 L714 L715 L716 L717 | L718 L719 L720 L721 L722 L723 | L724 L725 L726 L727 L728 L729 | L730 L731 L732 L733 L734 L735 | L736 L737 L738 L739 L740 L741 | L742 L743 L744 L745 L746 L747 | L748 L749 L750 L751 L752 L753 | L754 L755 L756 L757 L758 L759 | L760 L761 L762 L763 L764 L765 | L766 L767 L768 L769 L770 L771 | L772 L773 L774 L775 L776 L777 | L778 L779 L780 L781 L782 L783 | L784 L785 L786 L787 L788 L789 | L790 L791 L792 L793 L794 L795 | L796 L797 L798 L799 L800 L801 | L802 L803 L804 L805 L806 L807 | L808 L809 L810 L811 L812 L813 | L814 L815 L816 L817 L818 L819 | L820 L821 L822 L823 L824 L825 | L826 L827 L828 L829 L830 L831 | L832 L833 L834 L835 L836 L837 | L838 L839 L840 L841 L842 L843 | L844 L845 L846 L847 L848 L849 | L850 L851 L852 L853 L854 L855 | L856 L857 L858 L859 L860 L861 | L862 L863 L864 L865 L866 L867 | L868 L869 L870 L871 L872 L873 | L874 L875 L876 L877 L878 L879 | L880 L881 L882 L883 L884 L885 | L886 L887 L888 L889 L890 L891 | L892 L893 L894 L895 L896 L897 | L898 L899 L900 L901 L902 L903 | L904 L905 L906 L907 L908 L909 | L910 L911 L912 L913 L914 L915 | L916 L917 L918 L919 L920 L921 | L922 L923 L924 L925 L926 L927 | L928 L929 L930 L931 L932 L933 | L934 L935 L936 L937 L938 L939 | L940 L941 L942 L943 L944 L945 | L946 L947 L948 L949 L950 L951 | L952 L953 L954 L955 L956 L957 | L958 L959 L960 L961 L962 L963 | L964 L965 L966 L967 L968 L969 | L970 L971 L972 L973 L974 L975 | L976 L977 L978 L979 L980 L981 | L982 L983 L984 L985 L986 L987 | L988 L989 L990 L991 L992 L993 | L994 L995 L996 L997 L998 L999 | L1000 L1001 L1002 L1003 L1004 L1005 | L1006 L1007 L1008 L1009 L1010 L1011 | L1012 L1013 L1014 L1015 L1016 L1017 | L1018 L1019 L1020 L1021 L1022 L1023 | L1024 L1025 L1026 L1027 L1028 L1029 | L1030 L1031 L1032 L1033 L1034 L1035 | L1036 L1037 L1038 L1039 L1040 L1041 | L1042 L1043 L1044 L1045 L1046 L1047 | L1048 L1049 L1050 L1051 L1052 L1053 | L1054 L1055 L1056 L1057 L1058 L1059 | L1060 L1061 L1062 L1063 L1064 L1065 | L1066 L1067 L1068 L1069 L1070 L1071 | L1072 L1073 L1074 L1075 L1076 L1077 | L1078 L1079 L1080 L1081 L1082 L1083 | L1084 L1085 L1086 L1087 L1088 L1089 | L1090 L1091 L1092 L1093 L1094 L1095 | L1096 L1097 L1098 L1099 L1100 L1101 | L1102 L1103 L1104 L1105 L1106 L1107 | L1108 L1109 L1110 L1111 L1112 L1113 | L1114 L1115 L1116 L1117 L1118 L1119 | L1120 L1121 L1122 L1123 L1124 L1125 | L1126 L1127 L1128 L1129 L1130 L1131 | L1132 L1133 L1134 L1135 L1136 L1137 | L1138 L1139 L1140 L1141 L1142 L1143 | L1144 L1145 L1146 L1147 L1148 L1149 | L1150 L1151 L1152 L1153 L1154 L1155 | L1156 L1157 L1158 L1159 L1160 L1161 | L1162 L1163 L1164 L1165 L1166 L1167 | L1168 L1169 L1170 L1171 L1172 L1173 | L1174 L1175 L1176 L1177 L1178 L1179 | L1180 L1181 L1182 L1183 L1184 L1185 | L1186 L1187 L1188 L1189 L1190 L1191 | L1192 L1193 L1194 L1195 L1196 L1197 | L1198 L1199 L1200 L1201 L1202 L1203 | L1204 L1205 L1206 L1207 L1208 L1209 | L1210 L1211 L1212 L1213 L1214 L1215 | L1216 L1217 L1218 L1219 L1220 L1221 | L1222 L1223 L1224 L1225 L1226 L1227 | L1228 L1229 L1230 L1231 L1232 L1233 | L1234 L1235 L1236 L1237 L1238 L1239 | L1240 L1241 L1242 L1243 L1244 L1245 | L1246 L1247 L1248 L1249 L1250 L1251 | L1252 L1253 L1254 L1255 L1256 L1257 | L1258 L1259 L1260 L1261 L1262 L1263 | L1264 L1265 L1266 L1267 L1268 L1269 | L1270 L1271 L1272 L1273 L1274 L1275 | L1276 L1277 L1278 L1279 L1280 L1281 | L1282 L1283 L1284 L1285 L1286 L1287 | L1288 L1289 L1290 L1291 L1292 L1293 | L1294 L1295 L1296 L1297 L1298 L1299 | L1300 L1301 L1302 L1303 L1304 L1305 | L1306 L1307 L1308 L1309 L1310 L1311 | L1312 L1313 L1314 L1315 L1316 L1317 | L1318 L1319 L1320 L1321 L1322 L1323 | L1324 L1325 L1326 L1327 L1328 L1329 | L1330 L1331 L1332 L1333 L1334 L1335 | L1336 L1337 L1338 L1339 L1340 L1341 | L1342 L1343 L1344 L1345 L1346 L1347 | L1348 L1349 L1350 L1351 L1352 L1353 | L1354 L1355 L1356 L1357 L1358 L1359 | L1360 L1361 L1362 L1363 L1364 L1365 | L1366 L1367 L1368 L1369 L1370 L1371 | L1372 L1373 L1374 L1375 L1376 L1377 | L1378 L1379 L1380 L1381 L1382 L1383 | L1384 L1385 L1386 L1387 L1388 L1389 | L1390 L1391 L1392 L1393 L1394 L1395 | L1396 L1397 L1398 L1399 L1400 L1401 | L1402 L1403 L1404 L1405 L1406 L1407 | L1408 L1409 L1410 L1411 L1412 L1413 | L1414 L1415 L1416 L1417 L1418 L1419 | L1420 L1421 L1422 L1423 L1424 L1425 | L1426 L1427 L1428 L1429 L1430 L1431 | L1432 L1433 L1434 L1435 L1436 L1437 | L1438 L1439 L1440 L1441 L1442 L1443 | L1444 L1445 L1446 L1447 L1448 L1449 | L1450 L1451 L1452 L1453 L1454 L1455 | L1456 L1457 L1458 L1459 L1460 L1461 | L1462 L1463 L1464 L1465 L1466 L1467 | L1468 L1469 L1470 L1471 L1472 L1473 | L1474 L1475 L1476 L1477 L1478 L1479 | L1480 L1481 L1482 L1483 L1484 L1485